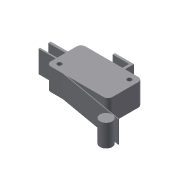
# Autodesk Inventor part: 00_Endstop
Saved by Autodesk Inventor 2019.4 (Build 234330000, 330)
## iProperties
Created: 2020-11-11
Part Number: 00_Endstop
Material: Generic
Document SubType Name: Modeling
Designer: diederichbenedict
Density: 1 g/cm^3
Appearance: Default
Author: diederichbenedict
Autodesk Inventor part; units mm, degrees
note: some values were not read from the file. Chosen so that the rebuilt part matches the saved one: sketch regions of "Extrusion1".
ref_plane "YZ Plane" through (0, 0, 0) normal (1, 0, 0) x (0, 1, 0)
ref_plane "XZ Plane" through (0, 0, 0) normal (0, 1, 0) x (-1, 0, 0)
ref_plane "XY Plane" through (0, 0, 0) normal (0, 0, 1) x (1, 0, 0)
sketch "Sketch1" plane through (0, 0, 0) normal (0, 1, 0) x (-1, 0, 0)
  line L0 (2, 0) -> (25.85, 0)
  line L1 (27.85, 2) -> (27.85, 13.7)
  line L2 (25.85, 15.7) -> (2, 15.7)
  line L3 (0, 13.7) -> (0, 2)
  arc A0 (27.85, 13.7) -> (25.85, 15.7) centre (25.85, 13.7) ccw
  arc A1 (25.85, 0) -> (27.85, 2) centre (25.85, 2) ccw
  arc A2 (0, 2) -> (2, 0) centre (2, 2) ccw
  arc A3 (2, 15.7) -> (0, 13.7) centre (2, 13.7) ccw
  line L4 (20.3653, 15.7) -> (-9.9478, 21.045)
  line L5 (18.6331, 15.7) -> (-10, 20.7488)
  line L6 (-10, 20.7488) -> (-9.9478, 21.045)
  circle A4 centre (-6.737, 23.2807) radius 2.7592
  circle A5 centre (24.85, 12.7) radius 1
  circle A6 centre (3, 3) radius 1
  point P0 (0, 0)
  point P1 (27.85, 15.7)
  point P2 (27.85, 0)
  point P3 (0, 15.7)
  dimension "d0" = 27.85
  dimension "d1" = 15.7
  dimension "d2" = 2
  dimension "d5" = 170
  dimension "d6" = 10
  dimension "d7" = 2
  dimension "d8" = 2
  dimension "d9" = 3
  dimension "d10" = 3
  dimension "d11" = 3
  dimension "d12" = 3
  constraints: 14 end point, 11 point on line, 9 tangent, 8 point on circle, 7 centre point, 3 equal radius, 3 parallel, 2 perpendicular, 1 horizontal
  measures "d0" distance of point (0, 15.7) point (27.85, 15.7)
  measures "d1" distance of point (27.85, 15.7) point (27.85, 0)
  measures "d2" radius of A0
  measures "d5" angle of L2 L5
  measures "d6" distance from line of L3 L5.end
  measures "d7" diameter of A5
  measures "d8" diameter of A6
  measures "d9" distance from line of A6.centre L3
  measures "d10" distance from line of A6.centre L0
  measures "d11" distance from line of L2 A5.centre
  measures "d12" distance from line of A5.centre L1
extrude "Extrusion1" add sketch "Sketch1" along normal blind 10
sketch "Sketch2" plane through (0, 10, 0) normal (0, 1, 0) x (1, 0, 0)
  line L0 (-27.85, -2) -> (-27.85, -13.7) projected
  line L1 (-35.5947, -11.431) -> (-27.85, -11.431)
  line L2 (-27.85, -11.431) -> (-27.85, -10.752)
  line L3 (-27.85, -10.752) -> (-35.5947, -10.752)
  line L4 (-35.5947, -10.752) -> (-35.5947, -11.431)
  line L5 (-35.5947, -7.0171) -> (-27.85, -7.0171)
  line L6 (-27.85, -7.0171) -> (-27.85, -5.9419)
  line L7 (-27.85, -5.9419) -> (-35.5947, -5.9419)
  line L8 (-35.5947, -5.9419) -> (-35.5947, -7.0171)
  line L9 (-16.5807, 2.9992) -> (-9.1675, 2.9992)
  line L10 (-9.1675, 2.9992) -> (-9.1675, 4.0178)
  line L11 (-9.1675, 4.0178) -> (-16.5807, 4.0178)
  line L12 (-16.5807, 4.0178) -> (-16.5807, 2.9992)
  line L13 (-9.1675, 4.0178) -> (-7.9791, 4.0178)
  line L14 (-7.9791, 4.0178) -> (-7.9791, 0)
  line L15 (-7.9791, 0) -> (-9.1675, 0)
  line L16 (-9.1675, 0) -> (-9.1675, 4.0178)
  point P0 (0, 0)
  constraints: 32 end point, 8 parallel, 4 horizontal, 4 perpendicular, 3 point on line
extrude "Extrusion2" add sketch "Sketch2" against normal up to surface (10 mm away)
body "Solid1"
